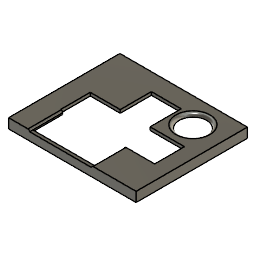
Top case (Autodesk Fusion 360 design; units mm, degrees)
part number: 2026-07-08-12-48-18-208
Autodesk Fusion 360 part; units mm, degrees
sketch "Sketch1" plane through (0, 0, 0) normal (0, 0, 1) x (1, 0, 0)
  line L0 (0, 0) -> (70.4, 0)
  line L1 (70.4, 0) -> (70.4, -60.4)
  line L2 (70.4, -60.4) -> (0, -60.4)
  line L3 (0, -60.4) -> (0, 0)
  dimension "d1" = 60.4
  dimension "d2" = 70.4
  constraint horizontal L0
  constraint vertical L1
  constraint horizontal L2
  constraint vertical L3
  constraint coincident L0.start L3.end
  measures "d1" distance of L0.start L2.end
  measures "d2" distance of L1 L3
extrude "Extrude1" add sketch "Sketch1" along normal blind 2
sketch "Sketch3" plane through (0, 0, 2) normal (0, 0, 1) x (-1, 0, 0)
  line L0 (0, 60.4) -> (-70.4, 60.4)
  line L1 (-70.4, 60.4) -> (-70.4, 0)
  line L2 (-70.4, 0) -> (0, 0)
  line L3 (0, 0) -> (0, 60.4)
  line L4 (-7.55, 25.79) -> (-65.55, 25.79)
  line L5 (-65.55, 25.79) -> (-65.55, 44.11)
  line L6 (-65.55, 44.11) -> (-7.55, 44.11)
  line L7 (-7.55, 44.11) -> (-7.55, 25.79)
  line L8 (-26, 25.79) -> (-44.32, 25.79)
  line L9 (-44.32, 25.79) -> (-44.32, 6.6)
  line L10 (-44.32, 6.6) -> (-26, 6.6)
  line L11 (-26, 6.6) -> (-26, 25.79)
  line L12 (-46.9, 60.4) -> (-8.9, 60.4)
  line L13 (-8.9, 60.4) -> (-8.9, 44.11)
  line L14 (-8.9, 44.11) -> (-46.9, 44.11)
  line L15 (-46.9, 44.11) -> (-46.9, 60.4)
  dimension "d19" = 58
  dimension "d20" = 18.32
  dimension "d21" = 7.55
  dimension "d22" = 70.4
  dimension "d23" = 18.32
  dimension "d24" = 19.19
  dimension "d25" = 6.6
  dimension "d26" = 26
  dimension "d27" = 16.29
  dimension "d28" = 38
  dimension "d29" = 8.9
  constraint horizontal L4
  constraint vertical L5
  constraint horizontal L6
  constraint vertical L7
  constraint horizontal L8
  constraint vertical L9
  constraint horizontal L10
  constraint vertical L11
  constraint coincident L4 L8.start
  constraint horizontal L12
  constraint vertical L13
  constraint horizontal L14
  constraint vertical L15
  constraint coincident L0 L12.start
  measures "d19" distance of L4.start L4.end
  measures "d20" distance of L4.start L6.end
  measures "d21" distance of L3 L7
  measures "d22" distance of L1 L3
  measures "d23" distance of L8.start L8.end
  measures "d24" distance of L8.start L10.end
  measures "d25" distance of L2 L10
  measures "d26" distance of L3 L11
  measures "d27" distance of L0 L6
  measures "d28" distance of L12.start L12.end
  measures "d29" distance of L3 L13
extrude "Extrude2" cut sketch "Sketch3" against normal blind 2 contours L0 L6 L12 L13 L14 L15 | L4 L5 L6 L7 L8 L14 | L4 L8 L9 L10 L11
sketch "Sketch4" plane through (0, 0, 2) normal (0, 0, 1) x (-1, 0, 0)
  line L0 (-46.9, 44.11) -> (-46.9, 60.4)
  line L1 (-46.9, 60.4) -> (-70.4, 60.4)
  line L2 (-70.4, 60.4) -> (-70.4, 0)
  line L3 (-70.4, 0) -> (0, 0)
  line L4 (0, 0) -> (0, 60.4)
  line L5 (0, 60.4) -> (-8.9, 60.4)
  line L6 (-8.9, 60.4) -> (-8.9, 44.11)
  line L7 (-8.9, 44.11) -> (-7.55, 44.11)
  line L8 (-7.55, 44.11) -> (-7.55, 25.79)
  line L9 (-7.55, 25.79) -> (-26, 25.79)
  line L10 (-26, 25.79) -> (-26, 6.6)
  line L11 (-26, 6.6) -> (-44.32, 6.6)
  line L12 (-44.32, 6.6) -> (-44.32, 25.79)
  line L13 (-44.32, 25.79) -> (-65.55, 25.79)
  line L14 (-65.55, 25.79) -> (-65.55, 44.11)
  line L15 (-65.55, 44.11) -> (-46.9, 44.11)
  circle A0 centre (-56.45, 11.45) radius 8.5
  dimension "d32" = 17
  dimension "d33" = 13.95
  dimension "d34" = 11.45
  measures "d32" diameter of A0
  measures "d33" distance of L2 A0.centre
  measures "d34" distance of L3 A0.centre
extrude "Extrude3" cut sketch "Sketch4" against normal blind 2 contours A0
fillet "Fillet1" radius 1 2 edges at (8.9, -52.255, 2) (46.9, -52.255, 2)
fillet "Fillet2" radius 2 1 edges at (64.3748, -14.5237, 2)
extrude "Extrude4" add 1 faces at (55.0667, -60.4, 0.6667) along direction (0, -1, 0) blind 2
extrude "Extrude5" add 1 faces at (5.6, -60.4, 0.6667) along direction (0, -1, 0) blind 2
extrude "Extrude6" add 1 faces at (0, -41.6, 1.3333) along direction (-1, 0, 0) blind 2
extrude "Extrude7" add 1 faces at (46.2667, 0, 0.6667) along direction (0, 1, 0) blind 2
extrude "Extrude13" add 1 faces at (70.4, -40.9333, 0.6667) along direction (1, 0, 0) blind 2
extrude "Extrude14" add 2 faces at (4.9333, -62.4, 0.6667) (55.7333, -62.4, 0.6667) along direction (0, -1, 0) blind 2.1
extrude "Extrude15" add 1 faces at (72.4, -42.3333, 0.6667) along direction (1, 0, 0) blind 2.1
extrude "Extrude16" add 1 faces at (49, 2, 1.3333) along direction (0, 1, 0) blind 2.1
extrude "Extrude17" add 1 faces at (-2, -18.7667, 1.3333) along direction (-1, 0, 0) blind 2.1
sketch "Sketch6" plane through (0, 0, 0) normal (0, 0, -1) x (1, 0, 0)
  circle A0 centre (56.45, 11.45) radius 8.5
  line L0 (46.9, 64.5) -> (46.9, 44.11)
  line L1 (46.9, 44.11) -> (65.55, 44.11)
  line L2 (65.55, 44.11) -> (65.55, 25.79)
  line L3 (65.55, 25.79) -> (44.32, 25.79)
  line L4 (44.32, 25.79) -> (44.32, 6.6)
  line L5 (44.32, 6.6) -> (26, 6.6)
  line L6 (26, 6.6) -> (26, 25.79)
  line L7 (26, 25.79) -> (7.55, 25.79)
  line L8 (7.55, 25.79) -> (7.55, 44.11)
  line L9 (7.55, 44.11) -> (8.9, 44.11)
  line L10 (8.9, 44.11) -> (8.9, 64.5)
  line L11 (8.9, 64.5) -> (-4.1, 64.5)
  line L12 (-4.1, 64.5) -> (-4.1, -4.1)
  line L13 (-4.1, -4.1) -> (74.5, -4.1)
  line L14 (74.5, -4.1) -> (74.5, 64.5)
  line L15 (74.5, 64.5) -> (46.9, 64.5)
  line L16 (-4.1, -4.1) -> (74.5, -4.1)
  line L17 (74.5, -4.1) -> (74.5, -2.1)
  line L18 (74.5, -2.1) -> (-4.1, -2.1)
  line L19 (-4.1, -2.1) -> (-4.1, -4.1)
  line L20 (74.5, -4.1) -> (72.5, -4.1)
  line L21 (72.5, -4.1) -> (72.5, 64.5)
  line L22 (72.5, 64.5) -> (74.5, 64.5)
  line L23 (74.5, 64.5) -> (74.5, -4.1)
  line L24 (-4.1, 64.5) -> (-2.1, 64.5)
  line L25 (-2.1, 64.5) -> (-2.1, -4.1)
  line L26 (-2.1, -4.1) -> (-4.1, -4.1)
  line L27 (-4.1, -4.1) -> (-4.1, 64.5)
  line L28 (-4.1, 64.5) -> (8.9, 64.5)
  line L29 (8.9, 64.5) -> (8.9, 62.5)
  line L30 (8.9, 62.5) -> (-4.1, 62.5)
  line L31 (-4.1, 62.5) -> (-4.1, 64.5)
  line L32 (46.9, 64.5) -> (74.5, 64.5)
  line L33 (74.5, 64.5) -> (74.5, 62.5)
  line L34 (74.5, 62.5) -> (46.9, 62.5)
  line L35 (46.9, 62.5) -> (46.9, 64.5)
  dimension "d69" = 2
  dimension "d70" = 2
  dimension "d71" = 2
  dimension "d72" = 2
  dimension "d73" = 2
  constraint horizontal L16
  constraint vertical L17
  constraint horizontal L18
  constraint vertical L19
  constraint coincident L12.end L13.start
  constraint horizontal L20
  constraint vertical L21
  constraint horizontal L22
  constraint vertical L23
  constraint horizontal L24
  constraint vertical L25
  constraint horizontal L26
  constraint vertical L27
  constraint coincident L11.end L12.start
  constraint horizontal L28
  constraint vertical L29
  constraint horizontal L30
  constraint vertical L31
  constraint horizontal L32
  constraint vertical L33
  constraint horizontal L34
  constraint vertical L35
  constraint coincident L0.start L15.end
  measures "d69" distance of L12.end L18.end
  measures "d70" distance of L13.end L20.end
  measures "d71" distance of L11.end L24.end
  measures "d72" distance of L11.end L30.end
  measures "d73" distance of L0.start L34.end
extrude "Extrude18" add sketch "Sketch6" along normal blind 4 contours L0 L15 L21 L32 L34 L35 | L14 L15 L21 L22 L23 L32 L33 L34 | L14 L18 L21 L23 L34 | L13 L16 L18 L21 L25 | L13 L14 L16 L17 L18 L20 L21 L23 | L12 L13 L16 L18 L19 L25 L26 L27 | L12 L18 L25 L27 L30 | L11 L12 L24 L25 L27 L28 L30 L31 | L10 L11 L25 L28 L29 L30
sketch "Sketch7" plane through (8.9, 0, 0) normal (1, 0, 0) x (0, 1, 0)
  line L0 (-44.11, 1) -> (-64.5, 1)
  line L1 (-64.5, 1) -> (-64.5, -4)
  line L2 (-64.5, -4) -> (-62.5, -4)
  line L3 (-62.5, -4) -> (-62.5, 0)
  line L4 (-62.5, 0) -> (-44.11, 0)
  line L5 (-44.11, 0) -> (-44.11, 1)
  line L6 (-62.5, -4) -> (-64.5, -4)
  line L7 (-64.5, -4) -> (-64.5, 1)
  line L8 (-64.5, 1) -> (-62.5, 1)
  line L9 (-62.5, 1) -> (-62.5, -4)
  constraint horizontal L6
  constraint vertical L7
  constraint horizontal L8
  constraint vertical L9
  constraint coincident L0.end L1.start
  constraint coincident L2.end L3.start
extrude "Extrude19" add sketch "Sketch7" along normal blind 38 contours L0 L1 L2 L3 L6 L7 L8 L9
